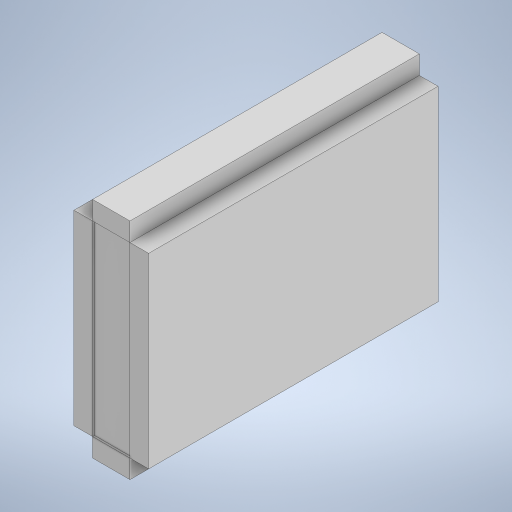
# Autodesk Inventor part: JukeBox CD Player
Saved by Autodesk Inventor 2024 (Build 280153000, 153)
## iProperties
Created: 2023-04-22
Part Number: JukeBox CD Player
Material: Generic
Document SubType Name: Modeling
Designer: newic
Density: 1 g/cm^3
Appearance: Default
Author: newic
Autodesk Inventor part; units mm, degrees
ref_plane "YZ Plane" through (0, 0, 0) normal (1, 0, 0) x (0, 1, 0)
ref_plane "XZ Plane" through (0, 0, 0) normal (0, 1, 0) x (-1, 0, 0)
ref_plane "XY Plane" through (0, 0, 0) normal (0, 0, 1) x (1, 0, 0)
sketch "Sketch1" plane through (0, 0, 0) normal (0, 0, 1) x (1, 0, 0)
  line L0 (0, 0) -> (812.8, 0) construction
  line L1 (812.8, 0) -> (812.8, -406.4) construction
  line L2 (812.8, -406.4) -> (0, -406.4) construction
  line L3 (0, -406.4) -> (0, 0) construction
  line L4 (0, 0) -> (406.4, 0)
  line L5 (406.4, 0) -> (406.4, -25.4)
  line L6 (406.4, -25.4) -> (0, -25.4)
  line L7 (0, -25.4) -> (0, 0)
  line L8 (406.4, -25.4) -> (381, -25.4)
  line L9 (381, -25.4) -> (381, -406.4)
  line L10 (381, -406.4) -> (406.4, -406.4)
  line L11 (406.4, -406.4) -> (406.4, -25.4)
  line L12 (381, -406.4) -> (0, -406.4)
  line L13 (0, -406.4) -> (0, -381)
  line L14 (0, -381) -> (381, -381)
  line L15 (381, -381) -> (381, -406.4)
  line L16 (0, -381) -> (25.4, -381)
  line L17 (25.4, -381) -> (25.4, -25.4)
  line L18 (25.4, -25.4) -> (0, -25.4)
  line L19 (0, -25.4) -> (0, -381)
  dimension "d1" = 812.8
  dimension "d5" = 406.4
  dimension "d6" = 25.4
  dimension "d7" = 25.4
  dimension "d8" = 381
  dimension "d9" = 381
  dimension "d10" = 25.4
  dimension "d11" = 25.4
  constraints: 32 end point, 8 parallel, 4 horizontal, 4 perpendicular, 1 point on line, 2 other
  measures "d1" distance of L1.end L2.end
  measures "d5" distance of L5.end L6.end
  measures "d6" distance of L4.end L5.end
  measures "d7" distance of L10.end L9.end
  measures "d8" distance of L9.end L8.end
  measures "d9" distance of L13.end L14.end
  measures "d10" distance of L12.end L13.end
  measures "d11" distance of L18.end L17.end
extrude "Extrusion1" add sketch "Sketch1" against normal blind 25.4 contours L6 L9 L14 L17
sketch "Sketch3" plane through (0, 0, 0) normal (0, 0, 1) x (1, 0, 0)
  line L0 (-406.4, 0) -> (406.4, 0) construction
  line L1 (406.4, 0) -> (406.4, -406.4) construction
  line L2 (406.4, -406.4) -> (-406.4, -406.4) construction
  line L3 (-406.4, -406.4) -> (-406.4, 0) construction
  line L4 (406.4, -406.4) -> (406.4, 0)
  line L5 (381, -381) -> (25.4, -381) projected
  line L6 (25.4, -381) -> (177.8, -381)
  line L7 (177.8, -381) -> (203.2, -381)
  line L8 (177.8, -381) -> (177.8, -355.6)
  line L9 (177.8, -355.6) -> (228.6, -355.6)
  line L10 (228.6, -355.6) -> (228.6, -330.2)
  line L11 (228.6, -330.2) -> (254, -330.2)
  line L12 (254, -330.2) -> (254, -76.2)
  line L13 (254, -76.2) -> (228.6, -76.2)
  line L14 (228.6, -76.2) -> (228.6, -50.8)
  line L15 (228.6, -50.8) -> (177.8, -50.8)
  line L16 (177.8, -50.8) -> (177.8, -76.2)
  line L17 (177.8, -76.2) -> (152.4, -76.2)
  line L18 (152.4, -76.2) -> (152.4, -330.2)
  line L19 (152.4, -330.2) -> (177.8, -330.2)
  line L20 (177.8, -330.2) -> (177.8, -355.6)
  point P0 (0, 0)
  dimension "d36" = 812.8
  dimension "d48" = 152.4
  dimension "d49" = 25.4
  dimension "d50" = 25.4
  dimension "d51" = 50.8
  dimension "d52" = 25.4
  dimension "d53" = 25.4
  dimension "d54" = 254
  dimension "d55" = 25.4
  dimension "d56" = 25.4
  dimension "d57" = 50.8
  dimension "d58" = 25.4
  dimension "d59" = 25.4
  dimension "d60" = 254
  dimension "d61" = 25.4
  constraints: 34 end point, 8 point on line, 5 perpendicular, 1 midpoint, 1 vertical, 2 other
  measures "d36" distance of L1.end L2.end
  measures "d48" distance of L5.end L6.end
  measures "d49" distance of L6.end L7.end
  measures "d50" distance of L6.end L8.end
  measures "d51" distance of L8.end L9.end
  measures "d52" distance of L9.end L10.end
  measures "d53" distance of L10.end L11.end
  measures "d54" distance of L11.end L12.end
  measures "d55" distance of L12.end L13.end
  measures "d56" distance of L13.end L14.end
  measures "d57" distance of L14.end L15.end
  measures "d58" distance of L15.end L16.end
  measures "d59" distance of L16.end L17.end
  measures "d60" distance of L17.end L18.end
  measures "d61" distance of L18.end L19.end
extrude "Extrusion3" add sketch "Sketch3" along normal blind 393.7
sketch "Sketch4" plane through (381, -381, 0) normal (1, 0, 0) x (0, 0, -1)
  line L0 (0, 355.6) -> (25.4, 355.6) projected
  line L1 (153.8842, -0.5875) -> (0, -0.5875)
  line L2 (0, -0.5875) -> (0, 355.6)
  line L3 (0, 355.6) -> (153.8842, 355.6)
  line L4 (153.8842, 355.6) -> (153.8842, -0.5875)
  point P0 (0, 381)
  constraints: 8 end point, 2 parallel, 1 horizontal, 1 perpendicular
extrude "Extrusion4" cut sketch "Sketch4" against normal blind 393.7
sketch "Sketch5" plane through (0, 0, 393.7) normal (0, 0, 1) x (1, 0, 0)
  line L0 (177.8, -50.8) -> (177.8, -76.2) projected
  line L1 (228.6, -355.6) -> (228.6, -330.2) projected
  line L2 (177.8, -76.2) -> (228.6, -76.2)
  line L3 (228.6, -76.2) -> (228.6, -330.2)
  line L4 (228.6, -330.2) -> (177.8, -330.2)
  line L5 (177.8, -330.2) -> (177.8, -76.2)
  point P0 (0, 0)
  constraints: 8 end point, 2 parallel, 1 horizontal, 1 perpendicular
extrude "Extrusion5" cut sketch "Sketch5" against normal blind 2.54
body "Solid1"
